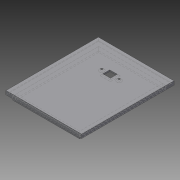
# Autodesk Inventor part: button_angle_top
Saved by Autodesk Inventor 2015 (Build 190159000, 159)
## iProperties
Created: 2014-10-13
Part Number: button_angle_top
Material: Generic
Document SubType Name: Modeling
Designer: Alec
Density: 1 g/cm^3
Appearance: Default
Author: Alec
Autodesk Inventor part; units mm, degrees
ref_plane "YZ Plane" through (0, 0, 0) normal (1, 0, 0) x (0, 1, 0)
ref_plane "XZ Plane" through (0, 0, 0) normal (0, 1, 0) x (-1, 0, 0)
ref_plane "XY Plane" through (0, 0, 0) normal (0, 0, 1) x (1, 0, 0)
sketch "Sketch1" plane through (0, 0, 0) normal (0, 1, 0) x (-1, 0, 0)
  line L0 (0, 0) -> (-114.3, 0)
  line L1 (-114.3, 0) -> (-114.3, -146.05)
  line L2 (-114.3, -146.05) -> (0, -146.05)
  line L3 (0, -146.05) -> (0, 0)
  dimension "d0" = 114.3
  dimension "d1" = 146.05
  constraints: 8 end point, 2 parallel, 1 horizontal, 1 perpendicular
  measures "d0" distance of L1.end L2.end
  measures "d1" distance of L0.end L1.end
extrude "Extrusion1" add sketch "Sketch1" against normal blind 6.35
sketch "Sketch2" plane through (0, 0, 0) normal (0, 1, 0) x (1, 0, 0)
  line L0 (-6.35, 151.892) -> (-6.35, -3.175)
  line L1 (0, 146.05) -> (0, 0) projected
  line L2 (-6.35, 151.892) -> (120.65, 151.892)
  line L3 (114.3, 146.05) -> (0, 146.05) projected
  line L4 (120.65, 151.892) -> (120.65, -3.175)
  line L5 (114.3, 0) -> (114.3, 146.05) projected
  line L6 (-6.35, -3.175) -> (120.65, -3.175)
  line L7 (0, 0) -> (114.3, 0) projected
  dimension "d5" = 6.35
  dimension "d6" = 5.842
  dimension "d7" = 6.35
  dimension "d8" = 3.175
  constraints: 8 end point, 2 horizontal, 2 vertical
  measures "d5" distance between parallel lines of L1 L0
  measures "d6" distance between parallel lines of L3 L2
  measures "d7" distance between parallel lines of L5 L4
  measures "d8" distance between parallel lines of L7 L6
extrude "Extrusion2" add sketch "Sketch2" along normal blind 6.35 contours L2 L4 L6 L0 | L3 L5 L7 L1
sketch "Sketch3" plane through (0, 6.35, 0) normal (0, 1, 0) x (1, 0, 0)
  line L0 (50.8, 113.792) -> (63.5, 113.792)
  line L1 (63.5, 113.792) -> (63.5, 102.362)
  line L2 (63.5, 102.362) -> (50.8, 102.362)
  line L3 (50.8, 102.362) -> (50.8, 113.792)
  circle A0 centre (42.545, 108.712) radius 1.5875
  circle A1 centre (71.755, 108.712) radius 1.5875
  line L4 (120.65, 151.892) -> (-6.35, 151.892) projected
  line L5 (-6.35, 151.892) -> (-6.35, -3.175) projected
  point P0 (0, 0)
  dimension "d11" = 12.7
  dimension "d12" = 11.43
  dimension "d13" = 3.175
  dimension "d14" = 3.175
  dimension "d15" = 8.255
  dimension "d16" = 8.255
  dimension "d19" = 38.1
  dimension "d20" = 57.15
  dimension "d21" = 6.35
  dimension "d22" = 6.35
  constraints: 8 end point, 2 centre point, 2 parallel, 1 horizontal, 1 perpendicular
  measures "d11" distance of L1.end L2.end
  measures "d12" distance of L0.end L1.end
  measures "d13" diameter of A0
  measures "d14" diameter of A1
  measures "d15" distance from line of A1.centre L1
  measures "d16" distance from line of A0.centre L3
  measures "d19" distance between parallel lines of L4 L0
  measures "d20" distance between parallel lines of L5 L3
  measures "d21" distance from line of L2 A1.centre
  measures "d22" distance from line of A0.centre L2
extrude "Extrusion3" cut sketch "Sketch3" against normal blind 25.4
sketch "Sketch4" plane through (0, -6.35, 0) normal (0, -1, 0) x (1, 0, 0)
  line L0 (0, 0) -> (114.3, 0)
  line L1 (114.3, 0) -> (114.3, -146.05)
  line L2 (114.3, -146.05) -> (0, -146.05)
  line L3 (0, -146.05) -> (0, 0)
  line L4 (1.016, -1.016) -> (113.284, -1.016)
  line L5 (113.284, -1.016) -> (113.284, -145.034)
  line L6 (113.284, -145.034) -> (1.016, -145.034)
  line L7 (1.016, -145.034) -> (1.016, -1.016)
  dimension "d27" = 1.016
  constraints: 16 end point, 4 parallel, 2 perpendicular, 1 horizontal, 3 other
  measures "d27" distance between parallel lines of L3 L7
extrude "Extrusion4" cut sketch "Sketch4" against normal blind 6.35
shell "Shell1" thickness 2.54 removed faces 1 at (59.2667, -6.35, -34.798)
sketch "Sketch5" plane through (0, -6.35, 0) normal (0, -1, 0) x (1, 0, 0)
  circle A0 centre (71.755, -108.712) radius 1.5875 projected
  circle A1 centre (71.755, -108.712) radius 4.1275
  circle A2 centre (42.545, -108.712) radius 1.5875 projected
  circle A3 centre (42.545, -108.712) radius 4.1275
  line L0 (66.04, -99.822) -> (48.26, -99.822)
  line L1 (48.26, -99.822) -> (48.26, -116.332)
  line L2 (48.26, -116.332) -> (66.04, -116.332)
  line L3 (66.04, -116.332) -> (66.04, -99.822)
  point P0 (0, 0)
  constraints: 8 end point, 2 centre point, 2 coincident, 2 parallel, 1 horizontal, 1 perpendicular
extrude "Extrusion5" cut sketch "Sketch5" against normal blind 10.3188
body "Solid1"
